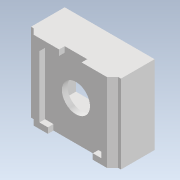
# Autodesk Inventor part: pid_test_structure
Saved by Autodesk Inventor 2020.2 (Build 242310000, 310)
## iProperties
Created: 2020-04-25
Part Number: pid_test_structure
Material: Generic
Document SubType Name: Modeling
Designer: Bardo91
Density: 1 g/cm^3
Appearance: Default
Author: Bardo91
Autodesk Inventor part; units mm, degrees
ref_plane "YZ Plane" through (0, 0, 0) normal (1, 0, 0) x (0, 1, 0)
ref_plane "XZ Plane" through (0, 0, 0) normal (0, 1, 0) x (-1, 0, 0)
ref_plane "XY Plane" through (0, 0, 0) normal (0, 0, 1) x (1, 0, 0)
sketch "Sketch1" plane through (0, 0, 0) normal (0, 0, 1) x (1, 0, 0)
  line L0 (-14.0621, 11.3836) -> (-2.0621, 11.3836)
  line L1 (-2.0621, 11.3836) -> (-2.0621, 1.3836)
  line L2 (-2.0621, 1.3836) -> (-14.0621, 1.3836)
  line L3 (-14.0621, 1.3836) -> (-14.0621, 11.3836)
  line L4 (-0.0621, 13.3836) -> (-16.0621, 13.3836)
  line L5 (-16.0621, 13.3836) -> (-16.0621, -0.6164)
  line L6 (-16.0621, -0.6164) -> (-0.0621, -0.6164)
  line L7 (-0.0621, -0.6164) -> (-0.0621, 13.3836)
  point P0 (0, 0)
  dimension "d0" = 12
  dimension "d1" = 10
  dimension "d2" = 2
  constraints: 16 end point, 4 parallel, 2 perpendicular, 1 horizontal, 3 other
  measures "d0" distance of L1.end L2.end
  measures "d1" distance of L0.end L1.end
  measures "d2" distance between parallel lines of L0 L4
extrude "Extrusion1" add sketch "Sketch1" against normal blind 5
sketch "Sketch2" plane through (0, 0, 0) normal (0, 0, 1) x (1, 0, 0)
  line L0 (-0.0621, 13.3836) -> (-16.0621, 13.3836) projected
  line L1 (-0.0621, -0.6164) -> (-0.0621, 13.3836) projected
  line L2 (-16.0621, 13.3836) -> (-0.0621, 13.3836)
  line L3 (-0.0621, 13.3836) -> (-0.0621, -0.6164)
  line L4 (-0.0621, -0.6164) -> (-16.0621, -0.6164)
  line L5 (-16.0621, -0.6164) -> (-16.0621, 13.3836)
  line L6 (-0.0621, 13.3836) -> (-0.0621, -0.6164) projected
  line L7 (-0.0621, 6.3836) -> (-16.0621, 6.3836)
  line L8 (-16.0621, -0.6164) -> (-16.0621, 13.3836) projected
  circle A0 centre (-8.0621, 6.3836) radius 2.5
  point P0 (0, 0)
  dimension "d7" = 5
  constraints: 10 end point, 3 midpoint, 2 parallel, 1 centre point, 1 horizontal, 1 perpendicular
  measures "d7" diameter of A0
extrude "Extrusion2" add sketch "Sketch2" along normal blind 1 contours L1 L7 A0 L5 L0 | L1 L4 L5 L7 A0
sketch "Sketch3" plane through (0, 0, 1) normal (0, 0, 1) x (1, 0, 0)
  line L0 (-13.5621, 12.3836) -> (-2.5621, 12.3836)
  line L1 (-2.5621, 12.3836) -> (-2.5621, 0.3836)
  line L2 (-2.5621, 0.3836) -> (-13.5621, 0.3836)
  line L3 (-13.5621, 0.3836) -> (-13.5621, 12.3836)
  line L4 (-8.0621, 12.3836) -> (-8.0621, 0.3836)
  circle A0 centre (-8.0621, 6.3836) radius 2.5 projected
  line L5 (-1.5621, 13.3836) -> (-14.5621, 13.3836)
  line L6 (-14.5621, 13.3836) -> (-14.5621, -0.6164)
  line L7 (-14.5621, -0.6164) -> (-1.5621, -0.6164)
  line L8 (-1.5621, -0.6164) -> (-1.5621, 13.3836)
  line L9 (-8.0621, 12.3836) -> (-10.0621, 12.3836)
  line L10 (-10.0621, 12.3836) -> (-10.0621, 13.3836)
  line L11 (-16.0621, 13.3836) -> (-0.0621, 13.3836) projected
  line L12 (-8.0621, 12.3836) -> (-6.0621, 12.3836)
  line L13 (-6.0621, 12.3836) -> (-6.0621, 13.3836)
  line L14 (-8.0621, 0.3836) -> (-4.0621, 0.3836)
  line L15 (-4.0621, 0.3836) -> (-4.0621, -0.6164)
  line L16 (-0.0621, -0.6164) -> (-16.0621, -0.6164) projected
  line L17 (-8.0621, 0.3836) -> (-12.0621, 0.3836)
  line L18 (-12.0621, 0.3836) -> (-12.0621, -0.6164)
  line L19 (-13.5621, 0.3836) -> (-13.5621, -0.6164)
  line L20 (-2.5621, 0.3836) -> (-2.5621, -0.6164)
  point P0 (0, 0)
  dimension "d8" = 11
  dimension "d9" = 12
  dimension "d10" = 1
  dimension "d11" = 2
  dimension "d12" = 2
  dimension "d13" = 4
  dimension "d14" = 4
  constraints: 38 end point, 10 point on line, 8 perpendicular, 4 parallel, 3 midpoint, 2 coincident, 1 horizontal, 3 other
  measures "d8" distance of L1.end L2.end
  measures "d9" distance of L0.end L1.end
  measures "d10" distance between parallel lines of L0 L5
  measures "d11" distance of L4.start L9.end
  measures "d12" distance of L4.start L12.end
  measures "d13" distance of L4.end L14.end
  measures "d14" distance of L4.end L17.end
extrude "Extrusion3" add sketch "Sketch3" along normal blind 1 contours L3 L19 L7 L6 L5 L10 L0 | L13 L5 L8 L7 L20 L1 L0
chamfer "Chamfer1" distance 1 angle 45 2 edges at (-14.5621, 6.3836, 1) (-1.5621, 6.3836, 1)
chamfer "Chamfer2" distance 3 angle 45 2 edges at (-13.5621, 12.3836, 1.5) (-2.5621, 12.3836, 1.5)
sketch "Sketch4" plane through (0, 0, 1) normal (0, 0, 1) x (1, 0, 0)
  circle A0 centre (-12.5621, 0.8836) radius 0.6
  circle A1 centre (-3.5621, 0.8836) radius 0.6
  line L0 (-12.5621, 0.8836) -> (-3.5621, 0.8836)
  circle A2 centre (-8.0621, 6.3836) radius 2.5 projected
  line L1 (-8.0621, 0.8836) -> (-8.0621, 6.3836)
  point P0 (0, 0)
  dimension "d23" = 1.2
  dimension "d24" = 1.2
  dimension "d25" = 5.5
  dimension "d26" = 9
  constraints: 4 end point, 2 centre point, 1 horizontal, 1 midpoint, 1 perpendicular
  measures "d23" diameter of A0
  measures "d24" diameter of A1
  measures "d25" distance of L1.start L1.end
  measures "d26" distance of L0.start L0.end
extrude "Extrusion4" cut sketch "Sketch4" against normal blind 2 contours A0 | A1
body "Solid1"
